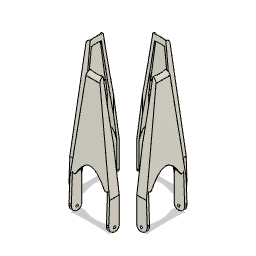
Rocket_Assembly_New_1 v6 (Autodesk Fusion 360 archive; units mm, degrees)
design "Landing_Legs"
Autodesk Fusion 360 part; units mm, degrees
sketch "Sketch14" plane through (22.5, 0, 0) normal (1, 0, 0) x (0, 0, -1)
  circle A0 centre (-42.5986, 7) radius 1.5
  arc A1 (-48.4364, 3) -> (-45.5175, 0.0011) centre (-45.4364, 3) ccw
  line L0 (-45.5175, 0.0011) -> (-45.5175, 2)
  line L1 (-36.7608, 2) -> (-36.7608, 12)
  line L2 (-36.7608, 12) -> (-43.4364, 12)
  arc A2 (-43.4364, 12) -> (-48.4364, 7) centre (-43.4364, 7) ccw
  line L3 (-48.4364, 7) -> (-48.4364, 3)
  line L4 (-41.9523, 2) -> (-27.3631, 2)
  line L5 (-43.4364, 11) -> (-37.7608, 11) construction
  line L6 (-37.7608, 11) -> (-37.7608, 2) construction
  line L7 (-41.9523, 3) -> (-27.3631, 3) construction
  line L8 (-37.7608, 11) -> (-37.7608, 3)
  line L9 (-50.0986, 12) -> (-50.0986, 10)
  line L10 (-42.0986, 2) -> (-41.7608, 2)
  line L11 (-35.0986, 12) -> (-50.0986, 2) construction
  line L12 (-50.0986, 12) -> (-35.0986, 2) construction
  arc A3 (-50.0986, 10) -> (-42.0986, 2) centre (-42.0986, 10) ccw
  line L13 (-36.7608, 12) -> (-36.7608, 2)
  line L14 (-36.7608, 7) -> (-36.7608, 12)
  arc A4 (-41.7608, 2) -> (-36.7608, 7) centre (-41.7608, 7) ccw
  line L15 (-36.7608, 12) -> (-36.7608, 164.4)
  line L16 (-36.7608, 164.4) -> (-39.9329, 164.4)
  line L17 (-44.9298, 159.575) -> (-50.0986, 12)
  arc A5 (-39.9329, 164.4) -> (-44.9298, 159.575) centre (-39.9329, 159.4) ccw
  point P0 (-42.5986, 7)
  point P1 (-44.7608, 164.4)
  dimension "d104" = -1
  dimension "d105" = 15
  dimension "d106" = 10
  dimension "d107" = 8
  dimension "d108" = 5
  dimension "d109" = 152.4
  dimension "d110" = 8
  dimension "d111" = 5
  constraint coincident L7 L8.end
  constraint coincident L6 L8.end
  constraint perpendicular L7 L8
  constraint coincident L11 P0
  constraint coincident L12 P0
  constraint coincident P0 A0.centre
  constraint coincident L11.end L9
  constraint coincident L11.end L10
  constraint tangent L9 A3
  constraint tangent L10 A3
  constraint coincident L1.end L2.start
  constraint coincident L1.start L10
  constraint tangent L10 A4
  constraint tangent L14 A4
  constraint perpendicular L2 L15
  constraint perpendicular L15 L16
  constraint coincident P1 L16
  constraint coincident P1 L17
  constraint tangent L16 A5
  constraint tangent L17 A5
  measures "d105" distance of L11.end L12.end
  measures "d106" distance of L9.start L11.end
  measures "d107" radius of A3
  measures "d108" radius of A4
  measures "d109" distance of L1.end L15.end
  measures "d110" distance of L15.end P1
  measures "d111" radius of A5
extrude "Extrude12" add sketch "Sketch14" along normal blind 3 contours L1 L2 A2 L3 L4 L10 A3 L13 L14 A4 | L2 A2 L3 L9 A3 L15 L16 L17 A5 makes body 1
mirror "Mirror1" about plane through (0, 0, 0) normal (1, 0, 0) of "Extrude12" makes body 2
sketch "Sketch15" plane through (22.5, 0, 0) normal (-1, 0, 0) x (0, 0, 1)
  circle A0 centre (42.5986, 7) radius 1.5
  arc A1 (44.9298, 159.575) -> (39.9329, 164.4) centre (39.9329, 159.4) ccw
  line L0 (39.9329, 164.4) -> (36.7608, 164.4)
  line L1 (36.7608, 164.4) -> (36.7608, 7)
  arc A2 (36.7608, 7) -> (41.7608, 2) centre (41.7608, 7) ccw
  line L2 (41.7608, 2) -> (42.0986, 2)
  arc A3 (42.0986, 2) -> (50.0986, 10) centre (42.0986, 10) ccw
  line L3 (50.0986, 10) -> (50.0986, 12)
  line L4 (50.0986, 12) -> (44.9298, 159.575)
  line L5 (42.5278, 40) -> (7, 40)
  line L6 (36.7608, 7) -> (36.7608, 164.4)
  line L7 (44.9298, 159.575) -> (50.0986, 12)
  arc A4 (44.9298, 159.575) -> (39.9329, 164.4) centre (39.9329, 159.4) ccw
  spline S0 degree 5 poles (36.7608, 40) (36.899, 40.8172) (37.184, 42.395) (37.6375, 44.5921) (38.2953, 47.1768) (39.2122, 49.7916) (40.2334, 51.7276) (41.3697, 52.9154) (42.63, 53.2964) (44.0152, 52.8649) (45.5183, 51.6663) (46.8087, 50.1362) (47.8229, 48.6865) (48.5193, 47.5879) (48.8726, 47.0056) knots 0 0 0 0 0 0 0.1 0.2 0.3 0.4 0.5 0.6 0.7 0.8 0.9 1 1 1 1 1 1
  line L8 (44.9298, 159.575) -> (48.8726, 47.0056)
  line L9 (36.7608, 7) -> (36.7608, 164.4)
  point P0 (42, 53)
  constraint coincident L5 S0.start
  constraint coincident L1 S0.start
  constraint coincident L4 S0.end
  constraint coincident A1.start L4.end
extrude "Extrude13" add sketch "Sketch15" along normal up to surface (45 mm away) contours A1 L0 L1 L4 L6 L7 A4 S0 L8 L9 bodies 1 2
sketch "Sketch16" plane through (0, 0, 36.7608) normal (0, 0, -1) x (-1, 0, 0)
  line L0 (22.5, 7) -> (25.5, 7)
  line L1 (25.5, 7) -> (25.5, 164.4)
  line L2 (25.5, 164.4) -> (-25.5, 164.4)
  line L3 (-25.5, 164.4) -> (-25.5, 7)
  line L4 (-25.5, 7) -> (-22.5, 7)
  line L5 (-22.5, 40) -> (22.5, 40)
  line L6 (0, 170) -> (0, 35) construction
  line L7 (-8.3333, 170) -> (-8.3333, 35) construction
  line L8 (-16.6667, 170) -> (-16.6667, 35) construction
  line L9 (-25, 170) -> (-25, 35) construction
  line L10 (-7, 40) -> (-42.5278, 40)
  line L11 (-25.5, 7) -> (-25.5, 164.4)
  line L12 (25.5, 164.4) -> (-25.5, 164.4)
  line L13 (25.5, 7) -> (25.5, 164.4)
  line L14 (42.5278, 40) -> (7, 40)
  line L15 (8.3333, 170) -> (8.3333, 35) construction
  line L16 (16.6667, 170) -> (16.6667, 35) construction
  line L17 (25, 170) -> (25, 35) construction
  line L18 (-25.5, 40) -> (-8.3333, 164.4)
  line L19 (8.3333, 164.4) -> (25.5, 40)
  line L20 (-22.5, 7) -> (-22.5, 40)
  line L21 (22.5, 40) -> (22.5, 7)
  dimension "d128" = -25
  dimension "d129" = 0
  dimension "d132" = 25
  dimension "d133" = 0
  constraint vertical L6
  constraint coincident L11 L18.start
  constraint coincident L10 L18.start
  constraint coincident L12 L18.end
  constraint coincident L7 L18.end
  constraint coincident L12 L19.start
  constraint coincident L15 L19.start
  constraint coincident L14 L19.end
  constraint coincident L1 L19.end
extrude "Extrude14" cut sketch "Sketch16" against normal blind 30 contours L1 L2 L12 L13 L19 | L2 L3 L11 L12 L18 bodies 1
sketch "Sketch17" plane through (0, 0, 36.7608) normal (0, 0, -1) x (-1, 0, 0)
  line L0 (25.5, 40) -> (8.3333, 164.4)
  line L1 (8.3333, 164.4) -> (-8.3333, 164.4)
  line L2 (-8.3333, 164.4) -> (-25.5, 40)
  line L3 (-25.5, 40) -> (-25.5, 7)
  line L4 (-25.5, 7) -> (-22.5, 7)
  line L5 (-22.5, 7) -> (-22.5, 40)
  line L6 (-22.5, 40) -> (22.5, 40)
  line L7 (22.5, 40) -> (22.5, 7)
  line L8 (22.5, 7) -> (25.5, 7)
  line L9 (25.5, 7) -> (25.5, 40)
  line L10 (-22.5, 40) -> (22.5, 40)
  spline S0 degree 5 poles (-22.5, 40) (-21.6, 41.8962) (-19.8, 45.523) (-17.1, 50.4664) (-13.5, 56.0476) (-9, 61.2265) (-4.5, 64.4472) (0, 65.5499) (4.5, 64.4472) (9, 61.2265) (13.5, 56.0476) (17.1, 50.4664) (19.8, 45.523) (21.6, 41.8962) (22.5, 40) knots 0 0 0 0 0 0 0.1 0.2 0.3 0.4 0.5 0.6 0.7 0.8 0.9 1 1 1 1 1 1
  point P0 (0, 65)
  constraint coincident L5.end L6.start
  constraint coincident L6.end L7.start
extrude "Extrude15" cut sketch "Sketch17" against normal blind 40 contours L6 L10 S0 bodies 1
sketch "Sketch18" plane through (0, 0, 36.7608) normal (0, 0, -1) x (-1, 0, 0)
  spline S0 degree 5 poles (-22.5, 40) (-21.6, 41.8962) (-19.8, 45.523) (-17.1, 50.4664) (-13.5, 56.0476) (-9, 61.2265) (-4.5, 64.4472) (0, 65.5499) (4.5, 64.4472) (9, 61.2265) (13.5, 56.0476) (17.1, 50.4664) (19.8, 45.523) (21.6, 41.8962) (22.5, 40) knots 0 0 0 0 0 0 0.1 0.2 0.3 0.4 0.5 0.6 0.7 0.8 0.9 1 1 1 1 1 1
  line L0 (22.5, 40) -> (22.5, 7)
  line L1 (22.5, 7) -> (25.5, 7)
  line L2 (25.5, 7) -> (25.5, 40)
  line L3 (25.5, 40) -> (8.3333, 164.4)
  line L4 (8.3333, 164.4) -> (-8.3333, 164.4)
  line L5 (-8.3333, 164.4) -> (-25.5, 40)
  line L6 (-25.5, 40) -> (-25.5, 7)
  line L7 (-25.5, 7) -> (-22.5, 7)
  line L8 (-22.5, 7) -> (-22.5, 40)
  line L9 (8.3333, 164.4) -> (-8.3333, 164.4)
  spline S1 degree 5 poles (-22.5, 40) (-21.6, 41.8962) (-19.8, 45.523) (-17.1, 50.4664) (-13.5, 56.0476) (-9, 61.2265) (-4.5, 64.4472) (0, 65.5499) (4.5, 64.4472) (9, 61.2265) (13.5, 56.0476) (17.1, 50.4664) (19.8, 45.523) (21.6, 41.8962) (22.5, 40) knots 0 0 0 0 0 0 0.1 0.2 0.3 0.4 0.5 0.6 0.7 0.8 0.9 1 1 1 1 1 1
  line L10 (-8.3333, 164.4) -> (-25.5, 40)
  line L11 (25.5, 40) -> (8.3333, 164.4)
  line L12 (1.5998, 159.6734) -> (-1.5998, 159.6734)
  line L13 (22.5282, 39.5899) -> (22.4599, 40.0844)
  line L14 (21.2227, 49.0501) -> (6.5528, 155.3569)
  line L15 (-6.5528, 155.3569) -> (-21.2202, 49.0682)
  line L16 (-22.4599, 40.0844) -> (-22.5282, 39.5899)
  arc A0 (-1.5998, 159.6734) -> (-6.5528, 155.3569) centre (-1.5998, 154.6734) ccw
  line L17 (22.5, 40) -> (21.2227, 49.0501)
  line L18 (-22.5, 40) -> (-21.2202, 49.0682)
  arc A1 (6.5528, 155.3569) -> (1.5998, 159.6734) centre (1.5998, 154.6734) ccw
  line L19 (-14.4501, 98.1288) -> (14.4501, 98.1288)
  line L20 (-9.7379, 132.2757) -> (9.7379, 132.2757)
  dimension "d148" = 5
  dimension "d149" = 5
  constraint parallel L11 L13
  constraint parallel L9 L12
  constraint parallel L10 L15
  constraint coincident S0 L13.end
  constraint collinear L13 L14
  constraint coincident S0 L16.start
  constraint collinear L15 L16
  constraint tangent L12 A0
  constraint tangent L15 A0
  constraint coincident S0.end L0.start
  constraint coincident S0.start L8.end
  constraint tangent L14 A1
  constraint tangent L12 A1
  constraint coincident L15 L19.start
  constraint coincident L14 L19.end
  constraint horizontal L19
  constraint coincident L15 L20.start
  constraint coincident L14 L20.end
  constraint parallel L19 L20
  measures "d148" radius of A0
  measures "d149" radius of A1
extrude "Extrude16" cut sketch "Sketch18" against normal blind 3 contours S0 S1 L14 L15 L17 L18 L19 | L14 L15 L19 L20 | L12 L14 L15 A0 A1 L20 bodies 1
sketch "Sketch20" plane through (0, 0, 39.7608) normal (0, 0, -1) x (-1, 0, 0)
  line L0 (20.9928, 50.7159) -> (16.7733, 50.7159)
  line L1 (20.9928, 50.7159) -> (6.5528, 155.3569)
  arc A0 (6.5528, 155.3569) -> (1.5998, 159.6734) centre (1.5998, 154.6734) ccw
  line L2 (1.5998, 159.6734) -> (-1.5998, 159.6734)
  arc A1 (-1.5998, 159.6734) -> (-6.5528, 155.3569) centre (-1.5998, 154.6734) ccw
  line L3 (-6.5528, 155.3569) -> (-20.9928, 50.7159)
  line L4 (-16.7733, 50.7159) -> (-20.9928, 50.7159)
  spline S0 degree 3 poles (16.7733, 50.7159) (15.1411, 53.3804) (13.4083, 55.8701) (10.0335, 59.8384) (8.1898, 61.667) (4.9595, 63.7606) (3.663, 64.3835) (1.0463, 65.0223) (-0.1931, 65.0823) (-2.9479, 64.6545) (-4.3557, 64.0735) (-7.7541, 62.0428) (-9.6485, 60.2336) (-13.1853, 56.1893) (-15.0364, 53.5514) (-16.7733, 50.7159) knots -6.172021 -6.172021 -6.172021 -6.172021 -5.231707 -5.231707 -4.417175 -4.417175 -3.939229 -3.939229 -3.513779 -3.513779 -3.004416 -3.004416 -2.184569 -2.184569 -1.193846 -1.193846 -1.193846 -1.193846
  line L5 (-15.3549, 91.5716) -> (-21.0078, 50.6074)
  line L6 (-16.8396, 50.6074) -> (-21.0078, 50.6074)
  spline S1 degree 3 poles (16.8396, 50.6074) (15.1881, 53.3128) (13.4329, 55.8413) (10.0335, 59.8384) (8.1898, 61.667) (4.9595, 63.7606) (3.663, 64.3835) (1.0463, 65.0223) (-0.1931, 65.0823) (-2.9479, 64.6545) (-4.3557, 64.0735) (-7.7541, 62.0428) (-9.6485, 60.2336) (-13.21, 56.1611) (-15.0835, 53.4841) (-16.8396, 50.6074) knots -6.18477 -6.18477 -6.18477 -6.18477 -5.231707 -5.231707 -4.417175 -4.417175 -3.939229 -3.939229 -3.513779 -3.513779 -3.004416 -3.004416 -2.184569 -2.184569 -1.181223 -1.181223 -1.181223 -1.181223
  line L7 (21.0078, 50.6074) -> (16.8396, 50.6074)
  line L8 (21.0078, 50.6074) -> (15.3549, 91.5716)
  line L9 (-15.3549, 91.5716) -> (15.3549, 91.5716)
  constraint coincident L3 L5.start
  constraint coincident L1 L8.end
  constraint horizontal L9
  constraint parallel L3 L5
  constraint parallel L4 L6
  constraint parallel L0 L7
  constraint parallel L1 L8
extrude "Extrude17" cut sketch "Sketch20" against normal blind 4 contours L0 L1 L3 L4 S0 L5 S1 L8 L9 bodies 1
sketch "Sketch21" plane through (0, 0, 39.7608) normal (0, 0, -1) x (-1, 0, 0)
  line L0 (-15.3549, 91.5716) -> (15.3549, 91.5716)
  line L1 (15.3549, 91.5716) -> (6.5528, 155.3569)
  arc A0 (6.5528, 155.3569) -> (1.5998, 159.6734) centre (1.5998, 154.6734) ccw
  line L2 (1.5998, 159.6734) -> (-1.5998, 159.6734)
  arc A1 (-1.5998, 159.6734) -> (-6.5528, 155.3569) centre (-1.5998, 154.6734) ccw
  line L3 (-6.5528, 155.3569) -> (-15.3549, 91.5716)
  line L4 (-11.7785, 117.4886) -> (-15.3549, 91.5716)
  line L5 (-15.3549, 91.5716) -> (15.3549, 91.5716)
  line L6 (15.3549, 91.5716) -> (11.7785, 117.4886)
  line L7 (-11.7785, 117.4886) -> (11.7785, 117.4886)
  constraint coincident L3 L4.start
  constraint coincident L1 L6.end
  constraint horizontal L7
  constraint parallel L3 L4
  constraint parallel L0 L5
  constraint parallel L1 L6
extrude "Extrude18" cut sketch "Sketch21" against normal blind 2 contours L0 L1 L3 L4 L5 L6 L7 bodies 1
fillet "Fillet11" radius 91.5 1 edges at (0, 91.5716, 43.7608) on bodies 1
fillet "Fillet12" radius 93.5 1 edges at (0, 117.4886, 41.7608) on bodies 1
fillet "Fillet13" radius 2.5 5 edges at (9.1656, 136.4227, 39.7608) (4.8848, 158.4429, 39.7608) (0, 159.6734, 39.7608) (-4.8848, 158.4429, 39.7608) (-9.1656, 136.4227, 39.7608) on bodies 1
sketch "Sketch22" plane through (0, 0, 0) normal (0, 1, 0) x (1, 0, 0)
  circle A0 centre (0, 0) radius 41
  dimension "d166" = 82
  constraint coincident A0.centre origin
  measures "d166" diameter of A0
ref_plane "WorkPlane3" through (0, 0, 35) normal (0, 0, 1) x (1, 0, 0)
sketch "Sketch26" plane through (0, 0, 35) normal (0, 0, 1) x (1, 0, 0)
  line L0 (-25.5, 40) -> (-8.9992, 159.575)
  line L1 (8.9992, 159.575) -> (-8.9992, 159.575)
  line L2 (8.9992, 159.575) -> (25.5, 40)
  line L3 (-12.8119, 110) -> (-6.3847, 156.575)
  line L4 (6.3847, 156.575) -> (-6.3847, 156.575)
  line L5 (6.3847, 156.575) -> (12.8119, 110)
  line L6 (0, 110) -> (-12.8119, 110)
  line L7 (0, 110) -> (12.8119, 110)
  constraint horizontal L6
  constraint parallel L6 L7
  constraint parallel L0 L3
  constraint parallel L1 L4
  constraint parallel L2 L5
extrude "Extrude20" cut sketch "Sketch26" along normal blind 7 bodies 1
pattern_circular "C-Pattern10" count 4 over 360 about axis through (0, 1.75, 0) along (0, 1, 0) of "Extrude12", "Mirror1", "Extrude13", "Extrude14", "Extrude15", "Extrude16", "Extrude17", "Extrude18", "Fillet11", "Fillet12", "Fillet13", "Extrude20" makes body 3 at (46.0341, 128.0478, 0.1174) makes body 4 at (0.1174, 128.0478, -46.0341) makes body 5 at (-46.0341, 128.0478, -0.1174)
sketch "Sketch27" plane through (0, 0, 0) normal (0, 1, 0) x (1, 0, 0)
  circle A0 centre (0, 0) radius 41
  dimension "d180" = 82
  constraint coincident A0.centre origin
  measures "d180" diameter of A0
extrude "Extrude21" cut sketch "Sketch27" along normal blind 270 bodies 1 3 4 5
named bodies: "Body15 (1)", "Body15 (2)", "Body15 (3)", "Body18 (1)", "Body18 (2)", "Body18 (3)"

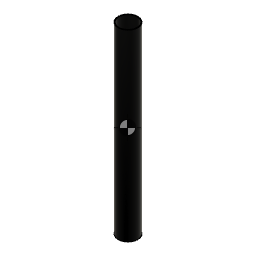
design "Rocket_Airframe_Tube"
Autodesk Fusion 360 part; units mm, degrees
sketch "Sketch1" plane through (0, 0, 0) normal (0, 1, 0) x (1, 0, 0)
  circle A0 centre (0, 0) radius 41
  circle A1 centre (0, 0) radius 38
  dimension "d1" = 82
  dimension "d2" = 76
  constraint coincident A0.centre A1.centre
  measures "d1" diameter of A0
  measures "d2" diameter of A1
extrude "Extrude1" add sketch "Sketch1" along normal blind 762

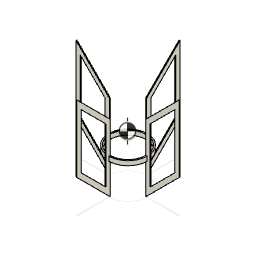
design "SIngle_Fin_2mm_Thickness_Square_Cuts"
Autodesk Fusion 360 part; units mm, degrees
sketch "Sketch1" plane through (0, 0, 0) normal (0, 1, 0) x (1, 0, 0)
  line L0 (1, 41.0878) -> (1, 117.3)
  line L1 (-1, 41.0878) -> (-1, 117.3)
  line L2 (-1, 117.3) -> (1, 117.3)
  arc A0 (1, 41.0878) -> (-1, 41.0878) centre (0, 0) ccw
  constraint coincident A0.centre origin
  constraint perpendicular L0 L2
extrude "Extrude1" add sketch "Sketch1" along normal blind 152.4 makes body 1
sketch "Sketch2" plane through (1, 0, 0) normal (1, 0, 0) x (0, 0, -1)
  line L0 (41.0878, 0) -> (117.3, 0)
  line L1 (117.3, 0) -> (117.3, 152.4)
  line L2 (117.3, 152.4) -> (41.0878, 152.4)
  line L3 (41.0878, 152.4) -> (41.0878, 0)
  line L4 (41.0878, 0) -> (117.3, 76.2122)
  line L5 (41.0878, 0) -> (148.8681, 0) construction
  line L6 (117.3, 0) -> (41.0878, 0)
  line L7 (117.3, 0) -> (117.3, 3.3314)
  line L8 (117.3, 0) -> (117.3, 76.2122)
  dimension "d7" = 45
  constraint horizontal L5
  constraint coincident L0.start L3.end
  constraint coincident L1 L4.end
  constraint coincident L0.end L1.start
  constraint coincident L1 L7.end
  measures "d7" angle of L4 L5
extrude "Extrude2" cut sketch "Sketch2" against normal blind 10 contours L0 L1 L4 L6 L7 L8 bodies 1
sketch "Sketch3" plane through (1, 0, 0) normal (1, 0, 0) x (0, 0, -1)
  line L0 (41.0878, 0) -> (117.3, 76.2122)
  line L1 (117.3, 76.2122) -> (117.3, 152.4)
  line L2 (117.3, 152.4) -> (41.0878, 152.4)
  line L3 (41.0878, 152.4) -> (41.0878, 0)
  line L4 (41.0878, 152.4) -> (117.3, 228.6122)
  line L5 (41.0878, 152.4) -> (148.8681, 152.4) construction
  line L6 (117.3, 228.6122) -> (117.3, 152.4)
  line L7 (41.0878, 152.4) -> (117.3, 152.4)
  dimension "d10" = 45
  constraint horizontal L5
  constraint coincident L2.end L3.start
  constraint coincident L1.end L2.start
  constraint perpendicular L2 L6
  measures "d10" angle of L4 L5
extrude "Extrude3" add sketch "Sketch3" against normal blind 2 contours L2 L4 L6 L7 bodies 1
sketch "Sketch5" plane through (1, 0, 0) normal (1, 0, 0) x (0, 0, -1)
  line L0 (41.0878, 0) -> (117.3, 76.2122)
  line L1 (117.3, 76.2122) -> (117.3, 228.6122)
  line L2 (117.3, 228.6122) -> (41.0878, 152.4)
  line L3 (41.0878, 152.4) -> (41.0878, 0)
  line L4 (51.0878, 148.2579) -> (107.3, 204.47)
  line L5 (107.3, 80.3543) -> (107.3, 204.47)
  line L6 (107.3, 80.3543) -> (51.0878, 24.1421)
  line L7 (51.0878, 148.2579) -> (51.0878, 24.1421)
extrude "Extrude5" cut sketch "Sketch5" against normal blind 10 contours L4 L5 L6 L7 bodies 1
sketch "Sketch7" plane through (1, 0, 0) normal (1, 0, 0) x (0, 0, -1)
  line L0 (51.0878, 148.2579) -> (107.3, 204.47)
  line L1 (107.3, 204.47) -> (107.3, 80.3543)
  line L2 (107.3, 80.3543) -> (51.0878, 24.1421)
  line L3 (51.0878, 24.1421) -> (51.0878, 148.2579)
  line L4 (41.0878, 0) -> (117.3, 76.2122)
  line L5 (117.3, 76.2122) -> (117.3, 228.6122)
  line L6 (117.3, 228.6122) -> (41.0878, 152.4)
  line L7 (41.0878, 152.4) -> (41.0878, 0)
  line L8 (41.0878, 81.2) -> (41.0878, 76.2)
  line L9 (41.0878, 71.2) -> (44.0878, 71.2)
  line L10 (44.0878, 71.2) -> (44.0878, 81.2)
  line L11 (44.0878, 81.2) -> (41.0878, 81.2)
  line L12 (38.0878, 71.2) -> (44.0878, 81.2) construction
  line L13 (44.0878, 71.2) -> (38.0878, 81.2) construction
  line L14 (41.0878, 71.2) -> (41.0878, 76.2)
  point P0 (41.0878, 76.2)
  dimension "d49" = 6
  dimension "d50" = 10
  constraint midpoint L7 P0
  constraint horizontal L9
  constraint perpendicular L9 L10
  constraint parallel L9 L11
  constraint coincident L12 P0
  constraint coincident L13 P0
  constraint coincident P0 L8.end
  constraint coincident L7 L9.start
  measures "d49" distance of L10.end L13.end
  measures "d50" distance of L9.end L10.end
extrude "Extrude6" cut sketch "Sketch7" against normal blind 3 contours L7 L8 L9 L10 L11 L14 bodies 1
sketch "Sketch8" plane through (0, 71.2, 0) normal (0, 1, 0) x (-1, 0, 0)
  arc A0 (-1, -41.0878) -> (1, -41.0878) centre (0, 0) ccw
  line L0 (-1, -41.0878) -> (-1, -44.0878)
  line L1 (-1, -44.0878) -> (1, -44.0878)
  line L2 (1, -44.0878) -> (1, -41.0878)
  circle A1 centre (0, 0) radius 41.1
  circle A2 centre (0, 0) radius 44.1
  dimension "d53" = 82.2
  dimension "d54" = 3
  constraint concentric A0 A1
  measures "d53" diameter of A1
extrude "Extrude7" add sketch "Sketch8" along normal blind 10 contours A0 L0 L1 L2 A1 | L0 L2 A1 A2 | L1 A2 bodies 1
pattern_circular "C-Pattern1" count 4 over 360 about axis through (0, 1.75, 0) along (0, 1, 0) of "Extrude1", "Extrude2", "Extrude3", "Extrude5", "Extrude6" makes body 2 at (-113.9667, 169.7648, -1) makes body 3 at (-1, 169.7648, 113.9667) makes body 4 at (113.9667, 169.7648, 1)
